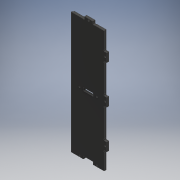
# Autodesk Inventor part: BA03
Saved by Autodesk Inventor 2017 (Build 210142000, 142)
## iProperties
Created: 2019-05-22
Part Number: BA03
Material: Polyethylene, High Density
Document SubType Name: Modeling
Designer: Dell
Density: 0.952 g/cm^3
Appearance: Smooth - Black
Mass: 197.966 g
Surface Area: 731.377 cm^2
Volume: 207.947 cm^3
Author: Dell
Autodesk Inventor part; units mm, degrees
ref_plane "YZ Plane" through (0, 0, 0) normal (1, 0, 0) x (0, 1, 0)
ref_plane "XZ Plane" through (0, 0, 0) normal (0, 1, 0) x (-1, 0, 0)
ref_plane "XY Plane" through (0, 0, 0) normal (0, 0, 1) x (1, 0, 0)
sketch "Sketch1" plane through (0, 0, 0) normal (0, 0, 1) x (1, 0, 0)
  line L0 (0, 0) -> (95.25, 0)
  line L1 (95.25, 0) -> (95.25, 6.35)
  line L2 (95.25, 6.35) -> (3.6662, 6.35)
  line L3 (3.6662, 6.35) -> (0, 0)
  dimension "d0" = 95.25
  dimension "d1" = 6.35
  dimension "d2" = 60
  constraints: 8 end point, 2 perpendicular, 1 horizontal
  measures "d0" distance of L0.start L0.end
  measures "d1" distance of L0.end L1.end
  measures "d2" angle of L0 L3
extrude "Extrusion1" add sketch "Sketch1" along normal blind 349.25
sketch "Sketch2" plane through (0, 0, 0) normal (0, -1, 0) x (1, 0, 0)
  line L0 (38.1, 349.25) -> (63.5, 349.25)
  line L1 (63.5, 349.25) -> (63.5, 355.6)
  line L2 (63.5, 355.6) -> (38.1, 355.6)
  line L3 (38.1, 355.6) -> (38.1, 349.25)
  line L4 (0, 349.25) -> (101.6, 349.25)
  line L5 (0, 349.25) -> (95.25, 349.25) projected
  point P0 (0, 0)
  point P1 (50.8, 349.25)
  dimension "d5" = 25.4
  dimension "d6" = 6.35
  dimension "d9" = 101.6
  constraints: 10 end point, 2 midpoint, 2 parallel, 1 collinear, 1 horizontal, 1 perpendicular
  measures "d5" distance of L2.end L1.end
  measures "d6" distance of L1.end L0.end
  measures "d9" distance of L4.start L4.end
extrude "Extrusion2" add sketch "Sketch2" against normal blind 6.35
sketch "Sketch3" plane through (0, 0, 0) normal (0, -1, 0) x (1, 0, 0)
  line L0 (63.5, 349.25) -> (63.5, 355.6) projected
  line L1 (63.5, 355.6) -> (38.1, 355.6) projected
  circle A0 centre (50.8, 352.425) radius 2.25
  point P0 (0, 0)
  point P1 (50.8, 355.6)
  point P2 (63.5, 352.425)
  dimension "d10" = 4.5
  constraints: 2 midpoint, 1 centre point, 1 horizontal alignment, 1 vertical alignment
  measures "d10" diameter of A0
extrude "Extrusion3" cut sketch "Sketch3" against normal through all
sketch "Sketch4" plane through (0, 0, 0) normal (0, -1, 0) x (1, 0, 0)
  line L0 (95.25, 0) -> (95.25, 349.25) projected
  line L1 (95.25, 50.8) -> (101.6, 50.8)
  line L2 (101.6, 50.8) -> (101.6, 76.2)
  line L3 (101.6, 76.2) -> (95.25, 76.2)
  line L4 (95.25, 76.2) -> (95.25, 50.8)
  line L5 (95.25, 298.45) -> (101.6, 298.45)
  line L6 (101.6, 298.45) -> (101.6, 273.05)
  line L7 (101.6, 273.05) -> (95.25, 273.05)
  line L8 (95.25, 273.05) -> (95.25, 298.45)
  line L9 (95.25, 187.325) -> (101.6, 187.325)
  line L10 (101.6, 187.325) -> (101.6, 161.925)
  line L11 (101.6, 161.925) -> (95.25, 161.925)
  line L12 (95.25, 161.925) -> (95.25, 187.325)
  circle A0 centre (98.425, 285.75) radius 2.25
  circle A1 centre (98.425, 174.625) radius 2.25
  circle A2 centre (98.425, 63.5) radius 2.25
  point P0 (0, 0)
  point P1 (95.25, 174.625)
  point P2 (98.425, 298.45)
  point P3 (98.425, 187.325)
  point P4 (98.425, 76.2)
  point P5 (101.6, 285.75)
  point P6 (101.6, 174.625)
  point P7 (101.6, 63.5)
  dimension "d14" = 25.4
  dimension "d15" = 6.35
  dimension "d16" = 25.4
  dimension "d18" = 25.4
  dimension "d19" = 50.8
  dimension "d20" = 50.8
  dimension "d21" = 4.5
  dimension "d22" = 4.5
  dimension "d23" = 4.5
  constraints: 24 end point, 8 midpoint, 6 parallel, 5 vertical alignment, 3 centre point, 3 horizontal, 3 horizontal alignment, 3 perpendicular, 3 point on line
  measures "d14" distance of L2.end L1.end
  measures "d15" distance of L6.end L7.end
  measures "d16" distance of L5.end L6.end
  measures "d18" distance of L9.end L10.end
  measures "d19" distance from line of L0.end L5
  measures "d20" distance from line of L0.start L1
  measures "d21" diameter of A0
  measures "d22" diameter of A1
  measures "d23" diameter of A2
extrude "Extrusion4" add sketch "Sketch4" against normal blind 6.35
sketch "Sketch6" plane through (95.25, 0, 298.45) normal (0, 0, 1) x (1, 0, 0)
  line L0 (-95.25, 0) -> (-84.2515, 6.35)
  line L1 (0, 6.35) -> (-91.5838, 6.35) projected
  line L2 (-95.25, 0) -> (0, 0) projected
  line L3 (-84.2515, 6.35) -> (-84.2515, 0)
  line L4 (-91.5838, 6.35) -> (-95.25, 0) projected
  line L5 (-84.2515, 6.35) -> (-84.2515, 6.35)
  line L6 (-84.2515, 6.35) -> (-91.5838, 6.35)
  dimension "d28" = 30
  dimension "d31" = 12.7
  constraints: 8 end point, 4 point on line, 1 collinear, 1 perpendicular, 1 vertical
  measures "d28" angle of L0 L2
  measures "d31" distance of L0.start L5.start
extrude "Extrusion6" [suppressed]
sketch "Sketch7" plane through (95.25, 0, 187.325) normal (0, 0, 1) x (1, 0, 0)
  line L0 (-77.9015, 12.7) -> (-77.9015, 6.35) projected
  line L1 (-81.5677, 12.7) -> (-77.9015, 12.7) projected
  line L2 (-88.9, 0) -> (-81.5677, 12.7) projected
  line L3 (-77.9015, 6.35) -> (-88.9, 0) projected
  point P0 (-95.25, 0)
extrude "Extrusion7" [suppressed]
sketch "Sketch8" plane through (95.25, 0, 76.2) normal (0, 0, 1) x (1, 0, 0)
  line L0 (-77.9015, 12.7) -> (-77.9015, 6.35) projected
  line L1 (-81.5677, 12.7) -> (-77.9015, 12.7) projected
  line L2 (-88.9, 0) -> (-81.5677, 12.7) projected
  line L3 (-77.9015, 6.35) -> (-88.9, 0) projected
  point P0 (-95.25, 0)
extrude "Extrusion8" [suppressed]
sketch "Sketch10" plane through (3.6662, 6.35, 0) normal (0, 1, 0) x (1, 0, 0)
  circle A0 centre (20.7919, -3.175) radius 2.25
  line L0 (90.648, -6.35) -> (0.9358, -6.35)
  circle A1 centre (70.7919, -3.175) radius 2.25
  line L1 (33.0919, -6.35) -> (58.4919, -6.35)
  line L2 (58.4919, -6.35) -> (58.4919, 0)
  line L3 (58.4919, 0) -> (33.0919, 0)
  line L4 (33.0919, 0) -> (33.0919, -6.35)
  line L5 (20.7919, -3.175) -> (70.7919, -3.175) construction
  line L6 (91.5838, 0) -> (0, 0) projected
  point P0 (-3.6662, 0)
  point P1 (45.7919, -3.175)
  point P2 (45.7919, -6.35)
  point P3 (45.7919, -6.35)
  point P4 (45.7919, 0)
  point P5 (33.0919, -3.175)
  dimension "d39" = 4.5
  dimension "d41" = 4.5
  dimension "d42" = 25.4
  dimension "d43" = 6.35
  dimension "d44" = 50
  constraints: 12 end point, 8 midpoint, 3 horizontal, 2 centre point, 2 parallel, 1 horizontal alignment, 1 perpendicular, 1 point on line, 1 vertical alignment
  measures "d39" diameter of A0
  measures "d41" diameter of A1
  measures "d42" distance of L3.end L2.end
  measures "d43" distance of L2.end L1.end
  measures "d44" distance of L5.start L5.end
extrude "Extrusion10" cut sketch "Sketch10" against normal through all
sketch "Sketch11" plane through (38.1, 0, 355.6) normal (0, -1, 0) x (1, 0, 0)
  line L0 (24.0581, -184.625) -> (-1.3419, -184.625)
  line L1 (-1.3419, -184.625) -> (-1.3419, -178.275)
  line L2 (-1.3419, -178.275) -> (24.0581, -178.275)
  line L3 (24.0581, -178.275) -> (24.0581, -184.625)
  line L4 (63.5, -168.275) -> (57.15, -168.275) projected
  line L5 (-1.3419, -349.25) -> (24.0581, -349.25) projected
  point P0 (-38.1, -355.6)
  point P1 (11.3581, -184.625)
  point P2 (11.3581, -349.25)
  dimension "d47" = 25.4
  dimension "d48" = 6.35
  dimension "d85" = 10
  constraints: 8 end point, 2 midpoint, 2 parallel, 1 horizontal, 1 perpendicular, 1 vertical alignment
  measures "d47" distance of L1.end L2.end
  measures "d48" distance of L0.end L1.end
  measures "d85" vertical distance of L2.end L4.start
extrude "Extrusion11" cut sketch "Sketch11" against normal through all
sketch "Sketch12" plane through (38.1, 0, 355.6) normal (0, -1, 0) x (1, 0, 0)
  circle A0 centre (-13.6419, -181.45) radius 2.25
  circle A1 centre (36.3581, -181.45) radius 2.25
  circle A2 centre (-13.6419, -352.425) radius 2.25 projected
  circle A3 centre (36.3581, -352.425) radius 2.25 projected
  line L0 (24.0581, -178.275) -> (24.0581, -184.625) projected
  point P0 (-38.1, -355.6)
  point P1 (24.0581, -181.45)
  dimension "d52" = 4.5
  dimension "d53" = 4.5
  constraints: 2 centre point, 2 horizontal alignment, 2 vertical alignment, 1 midpoint
  measures "d52" diameter of A0
  measures "d53" diameter of A1
extrude "Extrusion12" cut sketch "Sketch12" against normal through all contours A0 | A1
sketch "Sketch13" plane through (3.6662, 6.35, 349.25) normal (0, 1, 0) x (1, 0, 0)
  line L0 (58.4919, 349.25) -> (91.5838, 349.25) projected
  line L1 (59.7619, 349.25) -> (31.8219, 349.25)
  line L2 (31.8219, 349.25) -> (31.8219, 341.63)
  line L3 (31.8219, 341.63) -> (59.7619, 341.63)
  line L4 (59.7619, 341.63) -> (59.7619, 349.25)
  line L5 (59.7619, 179.545) -> (31.8219, 179.545)
  line L6 (31.8219, 179.545) -> (31.8219, 170.655)
  line L7 (31.8219, 170.655) -> (59.7619, 170.655)
  line L8 (59.7619, 170.655) -> (59.7619, 179.545)
  line L9 (58.4919, 342.9) -> (33.0919, 342.9) projected
  line L10 (33.0919, 178.275) -> (58.4919, 178.275) projected
  line L11 (58.4919, 178.275) -> (58.4919, 171.925) projected
  circle A0 centre (62.0789, -2.2451) radius 3.175
  circle A1 centre (32.1888, -2.2451) radius 3.175
  circle A2 centre (93.8289, 48.5549) radius 3.175
  circle A3 centre (93.8289, 78.4451) radius 3.175
  circle A4 centre (93.8289, 159.6799) radius 3.175
  circle A5 centre (93.8289, 189.5701) radius 3.175
  circle A6 centre (93.8289, 270.8049) radius 3.175
  circle A7 centre (93.8289, 300.6951) radius 3.175
  line L12 (97.9338, 298.45) -> (91.5838, 298.45) projected
  line L13 (91.5838, 298.45) -> (93.8289, 300.6951)
  line L14 (62.0789, -2.2451) -> (59.8338, 0) construction
  line L15 (59.8338, -6.35) -> (59.8338, 0) projected
  point P0 (-3.6662, 349.25)
  point P1 (45.7919, 342.9)
  point P2 (45.7919, 341.63)
  point P3 (45.7919, 178.275)
  point P4 (45.7919, 179.545)
  point P5 (58.4919, 175.1)
  point P6 (59.7619, 175.1)
  point P7 (91.5838, 273.05)
  point P8 (91.5838, 187.325)
  point P9 (91.5838, 161.925)
  point P10 (91.5838, 50.8)
  point P11 (91.5838, 76.2)
  point P12 (34.4338, 0)
  dimension "d61" = 6.35
  dimension "d62" = 6.35
  dimension "d63" = 6.35
  dimension "d64" = 6.35
  dimension "d65" = 6.35
  dimension "d66" = 6.35
  dimension "d67" = 6.35
  dimension "d68" = 6.35
  dimension "d56" = 1.27
  dimension "d57" = 1.27
  dimension "d58" = 1.27
  dimension "d69" = 45
  dimension "d70" = 45
  constraints: 20 end point, 9 vertical alignment, 6 midpoint, 4 parallel, 3 point on line, 2 horizontal, 2 horizontal alignment, 2 perpendicular, 1 coincident, 24 other
  measures "d56" distance between parallel lines of L3 L9
  measures "d57" distance between parallel lines of L8 L11
  measures "d58" distance between parallel lines of L5 L10
  measures "d69" angle of L12 L13
  measures "d70" angle of L15 L14
extrude "Extrusion13" cut sketch "Sketch13" against normal through all
sketch "Sketch14" plane through (3.6662, 6.35, 349.25) normal (0, 1, 0) x (1, 0, 0)
  line L0 (97.9338, 50.8) -> (96.074, 50.8) projected
  line L1 (97.9338, 50.8) -> (95.1652, 50.8)
  line L2 (95.1652, 50.8) -> (95.1652, 51.435)
  line L3 (95.1652, 51.435) -> (97.9338, 51.435)
  line L4 (97.9338, 51.435) -> (97.9338, 50.8)
  line L5 (97.9338, 50.8) -> (97.9338, 76.2) projected
  line L6 (97.9338, 76.2) -> (95.1652, 76.2)
  line L7 (95.1652, 76.2) -> (95.1652, 75.565)
  line L8 (95.1652, 75.565) -> (97.9338, 75.565)
  line L9 (97.9338, 75.565) -> (97.9338, 76.2)
  line L10 (97.9338, 161.925) -> (96.074, 161.925) projected
  line L11 (97.9338, 161.925) -> (95.1652, 161.925)
  line L12 (95.1652, 161.925) -> (95.1652, 162.56)
  line L13 (95.1652, 162.56) -> (97.9338, 162.56)
  line L14 (97.9338, 162.56) -> (97.9338, 161.925)
  line L15 (96.074, 187.325) -> (97.9338, 187.325) projected
  line L16 (97.9338, 187.325) -> (95.1652, 187.325)
  line L17 (95.1652, 187.325) -> (95.1652, 186.69)
  line L18 (95.1652, 186.69) -> (97.9338, 186.69)
  line L19 (97.9338, 186.69) -> (97.9338, 187.325)
  line L20 (97.9338, 273.05) -> (97.9338, 298.45) projected
  line L21 (97.9338, 273.05) -> (95.1652, 273.05)
  line L22 (95.1652, 273.05) -> (95.1652, 273.685)
  line L23 (95.1652, 273.685) -> (97.9338, 273.685)
  line L24 (97.9338, 273.685) -> (97.9338, 273.05)
  line L25 (97.9338, 298.45) -> (95.1652, 298.45)
  line L26 (95.1652, 298.45) -> (95.1652, 297.815)
  line L27 (95.1652, 297.815) -> (97.9338, 297.815)
  line L28 (97.9338, 297.815) -> (97.9338, 298.45)
  arc A0 (91.5838, 302.9401) -> (96.074, 298.45) centre (93.8289, 300.6951) ccw projected
  line L29 (34.4338, -6.35) -> (59.8338, -6.35) projected
  arc A1 (64.324, 0) -> (59.8338, -4.4901) centre (62.0789, -2.2451) ccw projected
  line L30 (59.8338, -6.35) -> (59.1988, -6.35)
  line L31 (59.1988, -6.35) -> (59.1988, -3.5814)
  line L32 (59.1988, -3.5814) -> (59.8338, -3.5814)
  line L33 (59.8338, -3.5814) -> (59.8338, -6.35)
  line L34 (34.4338, -4.4901) -> (34.4338, -6.35) projected
  arc A2 (34.4338, -4.4901) -> (29.9437, 0) centre (32.1888, -2.2451) ccw projected
  line L35 (34.4338, -6.35) -> (35.0688, -6.35)
  line L36 (35.0688, -6.35) -> (35.0688, -3.5814)
  line L37 (35.0688, -3.5814) -> (34.4338, -3.5814)
  line L38 (34.4338, -3.5814) -> (34.4338, -6.35)
  point P0 (-3.6662, 349.25)
  dimension "d71" = 0.635
  dimension "d72" = 0.635
  dimension "d73" = 0.635
  dimension "d74" = 0.635
  dimension "d75" = 0.635
  dimension "d76" = 0.635
  dimension "d77" = 0.635
  constraints: 64 end point, 16 parallel, 8 horizontal, 8 perpendicular, 5 point on line, 3 point on circle, 1 vertical alignment
  measures "d71" distance between parallel lines of L25 L27
  measures "d72" distance between parallel lines of L21 L23
  measures "d73" distance between parallel lines of L16 L18
  measures "d74" distance between parallel lines of L11 L13
  measures "d75" distance between parallel lines of L0 L3
  measures "d76" distance between parallel lines of L6 L8
  measures "d77" distance between parallel lines of L33 L31
extrude "Extrusion14" cut sketch "Sketch14" against normal through all
sketch "Sketch15" plane through (3.6662, 6.35, 349.25) normal (0, 1, 0) x (1, 0, 0)
  line L0 (97.9338, 273.685) -> (95.1652, 273.685) projected
  line L1 (97.9338, 273.685) -> (99.2038, 273.685)
  line L2 (99.2038, 273.685) -> (99.2038, 297.815)
  line L3 (99.2038, 297.815) -> (97.9338, 297.815)
  line L4 (97.9338, 297.815) -> (97.9338, 273.685)
  line L5 (97.9338, 186.69) -> (99.2038, 186.69)
  line L6 (99.2038, 186.69) -> (99.2038, 162.56)
  line L7 (99.2038, 162.56) -> (97.9338, 162.56)
  line L8 (97.9338, 162.56) -> (97.9338, 186.69)
  line L9 (97.9338, 51.435) -> (97.9338, 75.565) projected
  line L10 (97.9338, 75.565) -> (99.2038, 75.565)
  line L11 (99.2038, 75.565) -> (99.2038, 51.435)
  line L12 (99.2038, 51.435) -> (97.9338, 51.435)
  line L13 (97.9338, 51.435) -> (97.9338, 75.565)
  line L14 (35.0688, -6.35) -> (59.1988, -6.35) projected
  line L15 (59.1988, -6.35) -> (35.0688, -6.35)
  line L16 (35.0688, -6.35) -> (35.0688, -7.62)
  line L17 (35.0688, -7.62) -> (59.1988, -7.62)
  line L18 (59.1988, -7.62) -> (59.1988, -6.35)
  point P0 (-3.6662, 349.25)
  dimension "d80" = 1.27
  dimension "d81" = 1.27
  constraints: 32 end point, 8 parallel, 4 horizontal, 4 perpendicular, 3 coincident, 2 point on line, 1 vertical alignment
  measures "d80" distance of L2.end point (97.934, 297.815)
  measures "d81" distance of L17.end L14.end
extrude "Extrusion15" add sketch "Sketch15" against normal blind 6.35
equation "\"d1\" = Panel_Thickness"
equation "\"d6\" = Panel_Thickness"
equation "\"d7\" = Panel_Thickness"
equation "\"d15\" = Panel_Thickness"
equation "\"d24\" = Panel_Thickness"
equation "\"d43\" = Panel_Thickness"
equation "\"d48\" = Panel_Thickness"
equation "\"d61\" = d63"
equation "\"d62\" = d61"
equation "\"d63\" = d65"
equation "\"d64\" = d65"
equation "\"d65\" = d68"
equation "\"d66\" = d68"
equation "\"d67\" = d68"
equation "\"d68\" = Tool_Dia"
equation "\"d56\" = Fit_Tolerance"
equation "\"d57\" = Fit_Tolerance"
equation "\"d58\" = Fit_Tolerance"
equation "\"d71\" = 0.5 * Fit_Tolerance"
equation "\"d72\" = 0.5 * Fit_Tolerance"
equation "\"d73\" = 0.5 * Fit_Tolerance"
equation "\"d74\" = 0.5 * Fit_Tolerance"
equation "\"d75\" = 0.5 * Fit_Tolerance"
equation "\"d76\" = 0.5 * Fit_Tolerance"
equation "\"d77\" = 0.5 * Fit_Tolerance"
equation "\"d80\" = Fit_Tolerance"
equation "\"d81\" = Fit_Tolerance"
equation "\"d82\" = Panel_Thickness"
equation "\"Panel_Thickness\" = 6.35"
equation "\"Fit_Tolerance\" = 1.27"
equation "\"Tool_Dia\" = 6.35"
body "Solid1"
